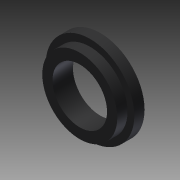
# Autodesk Inventor part: collar bearing systom
Saved by Autodesk Inventor 2012 (Build 160160000, 160)
## iProperties
Created: 2012-08-07
Part Number: collar bearing systom
Material: Default
Document SubType Name: Modeling
Designer: Bryce
Density: 1 g/cm^3
Author: Bryce
Autodesk Inventor part; units mm, degrees
ref_plane "YZ Plane" through (0, 0, 0) normal (1, 0, 0) x (0, 1, 0)
ref_plane "XZ Plane" through (0, 0, 0) normal (0, 1, 0) x (-1, 0, 0)
ref_plane "XY Plane" through (0, 0, 0) normal (0, 0, 1) x (1, 0, 0)
sketch "Sketch1" plane through (0, 0, 0) normal (0, 0, 1) x (1, 0, 0)
  circle A0 centre (0, 0) radius 12.7
  circle A1 centre (0, 0) radius 17.4625
  circle A2 centre (0, 0) radius 20.6375
  dimension "d0" = 25.4
  dimension "d1" = 34.925
  dimension "d2" = 41.275
  constraints: 3 centre point, 3 coincident
  measures "d0" diameter of A0
  measures "d1" diameter of A1
  measures "d2" diameter of A2
extrude "Extrusion1" add sketch "Sketch1" along normal blind 9.525 contours A1
extrude "Extrusion2" add sketch "Sketch1" along normal blind 4.7625 contours A2
body "Solid1"
